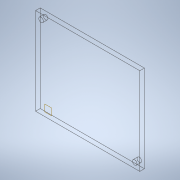
# Autodesk Inventor part: RelayTray
Saved by Autodesk Inventor 2022.2 (Build 262287000, 287)
## iProperties
Created: 2022-01-15
Part Number: RelayTray
Material: Generic
Document SubType Name: Modeling
Designer: siwat
Density: 1 g/cm^3
Appearance: Default
Author: siwat
Autodesk Inventor part; units mm, degrees
ref_plane "YZ Plane" through (0, 0, 0) normal (1, 0, 0) x (0, 1, 0)
ref_plane "XZ Plane" through (0, 0, 0) normal (0, 1, 0) x (-1, 0, 0)
ref_plane "XY Plane" through (0, 0, 0) normal (0, 0, 1) x (1, 0, 0)
ref_plane "Work Plane1" through (-62.4151, 1.9295, 0) normal (0, 0, 1) x (1, 0, 0)
sketch "Sketch1" plane through (-62.4151, 1.9295, 0) normal (0, 0, 1) x (1, 0, 0)
  line L0 (-5.0959, -1.798) -> (62.2123, -1.798)
  line L1 (62.2123, -1.798) -> (62.2123, 54.509)
  line L2 (62.2123, 54.509) -> (-5.0959, 54.509)
  line L3 (-5.0959, 54.509) -> (-5.0959, -1.798)
  circle A0 centre (58.9363, 1.5668) radius 1.5
  circle A1 centre (-1.5532, 51.0932) radius 1.5
  point P0 (62.4151, -1.9295)
  dimension "d0" = 3
  dimension "d1" = 3
  constraints: 8 end point, 2 centre point, 2 parallel, 1 horizontal, 1 perpendicular
  measures "d0" diameter of A0
  measures "d1" diameter of A1
extrude "Extrusion1" add sketch "Sketch1" along normal blind 3
body "Solid1"
